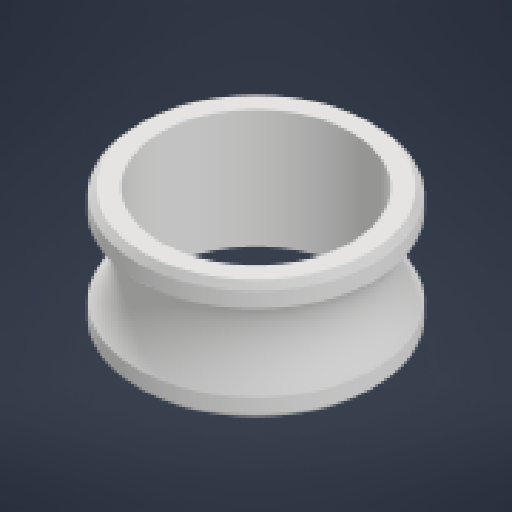
# Autodesk Inventor part: Inner_Ring
Saved by Autodesk Inventor 2023 (Build 270158000, 158)
## iProperties
Created: 2023-02-24
Part Number: Inner_Ring
Material: Generic
Document SubType Name: Modeling
Designer: izack
Density: 1 g/cm^3
Appearance: Default
di: 8.000 mm
p: 0.000 mm
Author: izack
Autodesk Inventor part; units mm, degrees
ref_plane "YZ Plane" through (0, 0, 0) normal (1, 0, 0) x (0, 1, 0)
ref_plane "XZ Plane" through (0, 0, 0) normal (0, 1, 0) x (-1, 0, 0)
ref_plane "XY Plane" through (0, 0, 0) normal (0, 0, 1) x (1, 0, 0)
sketch "Sketch1" plane through (0, 0, 0) normal (1, 0, 0) x (0, 1, 0)
  line L0 (0, 0) -> (7, 0)
  line L1 (0, 0) -> (0, -15) construction
  line L2 (0, -4) -> (5, -4)
  line L3 (5, -4) -> (5, -5)
  line L4 (5, -5) -> (0, -5)
  line L5 (0, -5) -> (0, -4)
  circle A0 centre (2.5, -6.4) radius 2.2
  line L6 (2.5, 0) -> (2.5, -6.4) construction
  point P0 (0.8029, -5)
  point P1 (4.1971, -5)
  dimension "d2" = 7
  dimension "d3" = 15
  dimension "d4" = 5
  dimension "d5" = 8
  dimension "d6" = 4.4
  dimension "d7" = 2.5
  dimension "d8" = 1.4
  dimension "d9" = 1
  constraints: 14 end point, 2 horizontal, 2 parallel, 2 point on line, 2 vertical, 1 centre point, 1 coincident, 1 perpendicular, 1 other
  measures "d2" distance of L0.start L0.end
  measures "d3" distance of L0.start L1.end
  measures "d4" distance of L3.end L4.end
  measures "d5" diameter of L2 L0
  measures "d6" diameter of A0
  measures "d7" distance between parallel lines of L1 L6
  measures "d8" distance from line of L4 L6.end
  measures "d9" distance between parallel lines of L2 L4
revolve "Revolution1" add sketch "Sketch1" angle 360 about axis through (0, 0, 0) along (0, 1, 0) contours L2 L3 L4 A0 L5
chamfer "Chamfer1" distance 0.25 angle 45 2 edges at (0, 5, 5) (0, 0, 5)
body "Solid1"
